Autodesk Fusion 360 part; units mm, degrees
(part 2 of 2)
sketch "Sketch4 (5)" plane through (0, 140, 0) normal (0, -1, 0) x (1, 0, 0) in component "Target holder left"
  line L0 (77, -34.8282) -> (74, -34.8282)
  line L1 (74, -34.8282) -> (74, -33.3282)
  line L2 (74, -33.3282) -> (77, -33.3282)
  line L3 (77, -33.3282) -> (77, -25.4282)
  line L4 (77, -25.4282) -> (62, -25.4282)
  line L5 (62, -25.4282) -> (62, -35.4282)
  line L6 (62, -35.4282) -> (77, -35.4282)
  line L7 (77, -35.4282) -> (77, -34.8282)
  line L8 (66.9731, -28.4282) -> (72.9731, -28.4282)
  line L9 (72.9731, -28.4282) -> (72.9731, -32.4282)
  line L10 (72.9731, -32.4282) -> (66.9731, -32.4282)
  line L11 (66.9731, -32.4282) -> (66.9731, -28.4282)
  line L12 (66.9731, -32.4282) -> (72.9731, -32.4282)
  line L13 (72.9731, -32.4282) -> (72.9731, -28.4282)
  line L14 (72.9731, -28.4282) -> (66.9731, -28.4282)
  line L15 (66.9731, -28.4282) -> (66.9731, -32.4282)
  constraint horizontal L12
  constraint vertical L13
  constraint horizontal L14
  constraint vertical L15
  constraint coincident L8.end L9.start
  constraint coincident L10.end L11.start
extrude "Extrude3''''''''" cut sketch "Sketch4 (5)" against normal blind 5 contours L8 L9 L10 L11 L12 L13 L14 L15 bodies 7 in component "Target holder left"
sketch "Sketch3 (8)" plane through (0, 140, 0) normal (0, -1, 0) x (1, 0, 0) in component "Target holder right"
  line L0 (243, -33.3282) -> (246, -33.3282)
  line L1 (246, -33.3282) -> (246, -34.8282)
  line L2 (246, -34.8282) -> (243, -34.8282)
  line L3 (243, -34.8282) -> (243, -35.4282)
  line L4 (243, -35.4282) -> (258, -35.4282)
  line L5 (258, -35.4282) -> (258, -25.4282)
  line L6 (258, -25.4282) -> (243, -25.4282)
  line L7 (243, -25.4282) -> (243, -33.3282)
  line L8 (246.9731, -28.4282) -> (252.9731, -28.4282)
  line L9 (252.9731, -28.4282) -> (252.9731, -32.4282)
  line L10 (252.9731, -32.4282) -> (246.9731, -32.4282)
  line L11 (246.9731, -32.4282) -> (246.9731, -28.4282)
  line L12 (246.9731, -28.4282) -> (252.9731, -28.4282)
  line L13 (252.9731, -28.4282) -> (252.9731, -32.4282)
  line L14 (252.9731, -32.4282) -> (246.9731, -32.4282)
  line L15 (246.9731, -32.4282) -> (246.9731, -28.4282)
  constraint horizontal L12
  constraint vertical L13
  constraint horizontal L14
  constraint vertical L15
  constraint coincident L9.end L10.start
  constraint coincident L8.start L11.end
extrude "Extrude3'''''''''" cut sketch "Sketch3 (8)" against normal blind 4 contours L8 L9 L10 L11 L12 L13 L14 L15 bodies 17 in component "Target holder right"
sketch "Sketch3 (9)" plane through (0, 0, -35.4282) normal (0, 0, -1) x (-1, 0, 0) in component "Target holder bottom"
  line L0 (-257.9731, 125.0758) -> (-61.9731, 125.0758)
  line L1 (-61.9731, 125.0758) -> (-61.9731, 140.0758)
  line L2 (-61.9731, 140.0758) -> (-257.9731, 140.0758)
  line L3 (-257.9731, 140.0758) -> (-257.9731, 125.0758)
  line L4 (-85.3026, 113.6358) -> (-67.6249, 131.3134)
  line L5 (-67.6249, 131.3134) -> (-77.5244, 141.2129)
  line L6 (-77.5244, 141.2129) -> (-95.2021, 123.5353)
  line L7 (-95.2021, 123.5353) -> (-85.3026, 113.6358)
  line L8 (-74.696, 138.3845) -> (-70.4534, 134.1419)
  line L9 (-70.4534, 134.1419) -> (-68.6856, 135.9096)
  line L10 (-68.6856, 135.9096) -> (-72.9282, 140.1523)
  line L11 (-72.9282, 140.1523) -> (-74.696, 138.3845)
  line L12 (-71.8676, 127.0708) -> (-81.06, 117.8784)
  line L13 (-81.06, 117.8784) -> (-79.2922, 116.1106)
  line L14 (-79.2922, 116.1106) -> (-70.0998, 125.303)
  line L15 (-70.0998, 125.303) -> (-71.8676, 127.0708)
  line L16 (-92.3737, 120.7068) -> (-88.131, 116.4642)
  line L17 (-88.131, 116.4642) -> (-89.8988, 114.6964)
  line L18 (-89.8988, 114.6964) -> (-94.1414, 118.9391)
  line L19 (-94.1414, 118.9391) -> (-92.3737, 120.7068)
  line L20 (-257.9731, 140.0758) -> (-257.9731, 125.0758)
  line L21 (-61.9731, 140.0758) -> (-257.9731, 140.0758)
  line L22 (-271.4131, 150.4053) -> (-253.7354, 132.7276)
  line L23 (-253.7354, 132.7276) -> (-243.8359, 142.6271)
  line L24 (-243.8359, 142.6271) -> (-261.5136, 160.3048)
  line L25 (-261.5136, 160.3048) -> (-271.4131, 150.4053)
  line L26 (-257.9731, 140.0758) -> (-257.9731, 136.9653)
  line L27 (-253.7354, 132.7276) -> (-257.9731, 136.9653)
  line L28 (-257.9731, 140.0758) -> (-246.3873, 140.0758)
  line L29 (-253.7354, 132.7276) -> (-246.3873, 140.0758)
  line L30 (-250.907, 135.5561) -> (-246.7408, 139.7222)
  line L31 (-246.7408, 139.7222) -> (-244.9731, 137.9545)
  line L32 (-244.9731, 137.9545) -> (-249.1392, 133.7883)
  line L33 (-249.1392, 133.7883) -> (-250.907, 135.5561)
  line L34 (-257.271, 136.2632) -> (-254.4425, 133.4348)
  line L35 (-254.4425, 133.4348) -> (-256.2103, 131.667)
  line L36 (-256.2103, 131.667) -> (-259.0387, 134.4954)
  line L37 (-259.0387, 134.4954) -> (-257.271, 136.2632)
  dimension "d197" = 2.5
  dimension "d198" = 2.5
  dimension "d199" = 2.5
  dimension "d200" = 4
  dimension "d201" = 4
  dimension "d202" = 6
  dimension "d203" = 6
  dimension "d204" = 4
  dimension "d205" = 4
  dimension "d221" = 2.5
  dimension "d222" = 4
  dimension "d223" = 0.5
  dimension "d238" = 2.5
  dimension "d239" = 1
  dimension "d240" = 4
  constraint perpendicular L8 L9
  constraint parallel L8 L10
  constraint parallel L9 L11
  constraint coincident L5 L8.end
  constraint coincident L5 L8.start
  constraint perpendicular L12 L13
  constraint parallel L12 L14
  constraint parallel L13 L15
  constraint coincident L4 L12.end
  constraint perpendicular L5 L12
  constraint perpendicular L16 L17
  constraint parallel L16 L18
  constraint parallel L17 L19
  constraint coincident L7 L16.end
  constraint perpendicular L14 L16
  constraint coincident L21 L28.end
  constraint coincident L23 L28.end
  constraint coincident L2.end L3.start
  constraint coincident L22 L26.end
  constraint coincident L20 L26.end
  constraint coincident L22.end L23.start
  constraint perpendicular L30 L31
  constraint parallel L30 L32
  constraint parallel L31 L33
  constraint coincident L23 L30.end
  constraint parallel L23 L30
  constraint perpendicular L34 L35
  constraint parallel L34 L36
  constraint parallel L35 L37
  constraint coincident L22 L34.end
  constraint parallel L22 L34
  measures "d197" distance of L8.end L9.end
  measures "d198" distance of L12.start L14.end
  measures "d199" distance of L16.end L17.end
  measures "d200" distance of L6.end L16.start
  measures "d201" distance of L4.start L16.end
  measures "d202" distance of L4.start L12.end
  measures "d203" distance of L4.end L12.start
  measures "d204" distance of L4.end L8.end
  measures "d205" distance of L5.end L8.start
  measures "d221" distance of L30.start L32.end
  measures "d222" distance of L22.end L30.start
  measures "d223" distance of L28.end L30.end
  measures "d238" distance of L34.end L35.end
  measures "d239" distance of L22.end L34.end
  measures "d240" distance of L34.start L34.end
extrude "Extrude8" add sketch "Sketch3 (9)" along normal blind 12 contours L0 L4 L12 L14 L15 | L0 L4 L12 L13 L14 | L7 L16 L17 L18 L19 | L2 L10 L11 L21 | L2 L5 L8 L9 L10 L11 L21 bodies 16 makes body 18 at (90.9595, 119.2926, -43.4282) in component "Target holder bottom"
extrude "Extrude10" add sketch "Sketch3 (9)" along normal blind 12 contours L3 L20 L22 L27 L34 L35 L36 L37 | L23 L29 L30 L31 L32 L33 bodies 16 in component "Target holder bottom"
extrude "Extrude11" add sketch "Sketch3 (9)" against normal blind 2 contours L0 L4 L6 L7 L12 L16 | L0 L4 L12 L13 L14 | L7 L16 L17 L18 L19 bodies 16 18 in component "Target holder bottom"
sketch "Sketch4 (6)" plane through (0, 0, -35.4282) normal (0, 0, -1) x (-1, 0, 0) in component "Target holder right"
  line L0 (-243, 310) -> (-258, 310)
  line L1 (-258, 310) -> (-258, 140)
  line L2 (-258, 140) -> (-243, 140)
  line L3 (-243, 140) -> (-243, 310)
  line L4 (-271.4131, 150.4053) -> (-253.7354, 132.7276)
  line L5 (-253.7354, 132.7276) -> (-243.8359, 142.6271)
  line L6 (-243.8359, 142.6271) -> (-261.5136, 160.3048)
  line L7 (-261.5136, 160.3048) -> (-271.4131, 150.4053)
  line L8 (-258, 156.7912) -> (-261.5136, 160.3048)
  line L9 (-261.5136, 160.3048) -> (-271.4131, 150.4053)
  line L10 (-258, 140) -> (-261.0078, 140)
  line L11 (-261.0078, 140) -> (-271.4131, 150.4053)
  line L12 (-258, 140) -> (-258, 156.7912)
  line L13 (-264.342, 157.4764) -> (-268.5847, 153.2337)
  line L14 (-268.5847, 153.2337) -> (-270.3524, 155.0015)
  line L15 (-270.3524, 155.0015) -> (-266.1098, 159.2442)
  line L16 (-266.1098, 159.2442) -> (-264.342, 157.4764)
  line L17 (-267.1705, 146.1627) -> (-261.3613, 140.3536)
  line L18 (-261.3613, 140.3536) -> (-263.1291, 138.5858)
  line L19 (-263.1291, 138.5858) -> (-268.9382, 144.3949)
  line L20 (-268.9382, 144.3949) -> (-267.1705, 146.1627)
  line L21 (-234.6436, 336.5158) -> (-252.3212, 318.8382)
  line L22 (-252.3212, 318.8382) -> (-242.4217, 308.9387)
  line L23 (-242.4217, 308.9387) -> (-224.7441, 326.6163)
  line L24 (-224.7441, 326.6163) -> (-234.6436, 336.5158)
  line L25 (-258, 310) -> (-252.3212, 318.8382)
  line L26 (-252.3212, 318.8382) -> (-234.6436, 336.5158)
  line L27 (-234.6436, 336.5158) -> (-224.7441, 326.6163)
  line L28 (-243, 310) -> (-241.3604, 310)
  line L29 (-241.3604, 310) -> (-224.7441, 326.6163)
  line L30 (-248.0786, 323.0808) -> (-238.8862, 332.2732)
  line L31 (-238.8862, 332.2732) -> (-240.654, 334.0409)
  line L32 (-240.654, 334.0409) -> (-249.8464, 324.8486)
  line L33 (-249.8464, 324.8486) -> (-248.0786, 323.0808)
  line L34 (-249.4928, 316.0097) -> (-245.2502, 311.7671)
  line L35 (-245.2502, 311.7671) -> (-247.0179, 309.9993)
  line L36 (-247.0179, 309.9993) -> (-251.2606, 314.242)
  line L37 (-251.2606, 314.242) -> (-249.4928, 316.0097)
  line L38 (-231.8151, 333.6874) -> (-227.5725, 329.4448)
  line L39 (-227.5725, 329.4448) -> (-225.8047, 331.2125)
  line L40 (-225.8047, 331.2125) -> (-230.0474, 335.4552)
  line L41 (-230.0474, 335.4552) -> (-231.8151, 333.6874)
  dimension "d228" = 2.5
  dimension "d229" = 2.5
  dimension "d230" = 4
  dimension "d231" = 4
  dimension "d232" = 6
  dimension "d233" = 0.5
  dimension "d254" = 2.5
  dimension "d255" = 6
  dimension "d256" = 6
  dimension "d257" = 2.5
  dimension "d258" = 4
  dimension "d259" = 4
  dimension "d261" = 2.5
  dimension "d262" = 4
  dimension "d263" = 4
  constraint coincident L1 L8.start
  constraint coincident L6 L8.start
  constraint coincident L6.end L7.start
  constraint coincident L4.start L7.end
  constraint coincident L1.end L2.start
  constraint coincident L4 L10.end
  constraint perpendicular L1 L10
  constraint perpendicular L13 L14
  constraint parallel L13 L15
  constraint parallel L14 L16
  constraint coincident L7 L13.end
  constraint parallel L7 L13
  constraint perpendicular L17 L18
  constraint parallel L17 L19
  constraint parallel L18 L20
  constraint coincident L11 L17.end
  constraint perpendicular L9 L17
  constraint coincident L0.end L1.start
  constraint coincident L21.end L22.start
  constraint coincident L21.start L24.end
  constraint coincident L23.end L24.start
  constraint coincident L0.start L3.end
  constraint coincident L23 L28.end
  constraint perpendicular L3 L28
  constraint perpendicular L30 L31
  constraint parallel L30 L32
  constraint parallel L31 L33
  constraint coincident L21 L30.end
  constraint parallel L21 L30
  constraint perpendicular L34 L35
  constraint parallel L34 L36
  constraint parallel L35 L37
  constraint coincident L22 L34.end
  constraint perpendicular L26 L34
  constraint perpendicular L38 L39
  constraint parallel L38 L40
  constraint parallel L39 L41
  constraint coincident L27 L38.end
  constraint perpendicular L35 L38
  measures "d228" distance of L13.end L14.end
  measures "d229" distance of L17.start L19.end
  measures "d230" distance of L4.start L13.end
  measures "d231" distance of L6.end L13.start
  measures "d232" distance of L4.start L17.start
  measures "d233" distance of L10.end L17.end
  measures "d254" distance of L30.start L32.end
  measures "d255" distance of L21.end L30.start
  measures "d256" distance of L21.start L30.end
  measures "d257" distance of L38.start L40.end
  measures "d258" distance of L21.start L38.start
  measures "d259" distance of L23.end L38.end
  measures "d261" distance of L34.start L36.end
  measures "d262" distance of L21.end L34.start
  measures "d263" distance of L22.end L34.end
extrude "Extrude4''''''''" add sketch "Sketch4 (6)" along normal blind 12 separate body contours L7 L9 L13 L14 L15 L16 | L4 L11 L17 L18 L19 L20 makes body 19 at (268.9382, 156.4157, -39.4282) makes body 20 at (265.2341, 144.2263, -39.4282) in component "Target holder right"
extrude "Extrude5'" add sketch "Sketch4 (6)" against normal blind 2 contours L1 L4 L6 L7 L8 L9 L10 L11 L12 L13 L17 | L7 L9 L13 L14 L15 L16 | L4 L11 L17 L18 L19 L20 bodies 17 19 20 in component "Target holder right"
sketch "Sketch5" plane through (0, 0, -35.4282) normal (0, 0, -1) x (-1, 0, 0) in component "Target holder left"
  line L0 (-62, 310) -> (-77, 310)
  line L1 (-77, 310) -> (-77, 140)
  line L2 (-77, 140) -> (-62, 140)
  line L3 (-62, 140) -> (-62, 310)
  line L4 (-48.533, 299.7463) -> (-66.2107, 317.4239)
  line L5 (-66.2107, 317.4239) -> (-76.1102, 307.5244)
  line L6 (-76.1102, 307.5244) -> (-58.4325, 289.8468)
  line L7 (-58.4325, 289.8468) -> (-48.533, 299.7463)
  line L8 (-73.2818, 310.3529) -> (-69.0391, 314.5955)
  line L9 (-69.0391, 314.5955) -> (-70.8069, 316.3633)
  line L10 (-70.8069, 316.3633) -> (-75.0496, 312.1206)
  line L11 (-75.0496, 312.1206) -> (-73.2818, 310.3529)
  line L12 (-61.9681, 313.1813) -> (-52.7757, 303.9889)
  line L13 (-52.7757, 303.9889) -> (-51.0079, 305.7567)
  line L14 (-51.0079, 305.7567) -> (-60.2003, 314.9491)
  line L15 (-60.2003, 314.9491) -> (-61.9681, 313.1813)
  line L16 (-51.3615, 296.9178) -> (-55.6041, 292.6752)
  line L17 (-55.6041, 292.6752) -> (-53.8364, 290.9074)
  line L18 (-53.8364, 290.9074) -> (-49.5937, 295.1501)
  line L19 (-49.5937, 295.1501) -> (-51.3615, 296.9178)
  line L20 (-66.2107, 317.4239) -> (-48.533, 299.7463)
  line L21 (-48.533, 299.7463) -> (-58.4325, 289.8468)
  line L22 (-58.4325, 289.8468) -> (-62, 293.4142)
  line L23 (-62, 293.4142) -> (-62, 310)
  line L24 (-73.6347, 310) -> (-73.2818, 310.3529)
  line L25 (-73.6347, 310) -> (-62, 310)
  dimension "d241" = 2.5
  dimension "d242" = 4
  dimension "d243" = 4
  dimension "d244" = 2.5
  dimension "d245" = 6
  dimension "d246" = 6
  dimension "d247" = 2.5
  dimension "d248" = 4
  dimension "d249" = 4
  constraint perpendicular L8 L9
  constraint parallel L8 L10
  constraint parallel L9 L11
  constraint coincident L5 L8.end
  constraint coincident L5 L8.start
  constraint perpendicular L12 L13
  constraint parallel L12 L14
  constraint parallel L13 L15
  constraint coincident L4 L12.end
  constraint perpendicular L5 L12
  constraint perpendicular L16 L17
  constraint parallel L16 L18
  constraint parallel L17 L19
  constraint coincident L7 L16.end
  constraint perpendicular L4 L16
  constraint coincident L4.end L5.start
  constraint coincident L4.start L7.end
  constraint coincident L6.end L7.start
  constraint coincident L3 L22.end
  constraint coincident L6 L22.end
  constraint coincident L0.start L3.end
  constraint coincident L0 L24.start
  constraint coincident L5 L24.start
  measures "d241" distance of L8.start L10.end
  measures "d242" distance of L5.end L8.start
  measures "d243" distance of L4.end L8.end
  measures "d244" distance of L12.start L14.end
  measures "d245" distance of L4.end L12.start
  measures "d246" distance of L4.start L12.end
  measures "d247" distance of L16.start L18.end
  measures "d248" distance of L4.start L16.start
  measures "d249" distance of L6.end L16.end
extrude "Extrude4'''''''''" add sketch "Sketch5" along normal blind 12 separate body contours L5 L8 L9 L10 L11 | L7 L16 L17 L18 L19 L21 | L4 L12 L13 L14 L15 L20 makes body 21 at (70.4534, 313.1813, -39.4282) makes body 22 at (54.0721, 308.8208, -39.4282) makes body 23 at (54.1899, 294.0894, -39.4282) in component "Target holder left"
extrude "Extrude5''" add sketch "Sketch5" against normal blind 2 contours L0 L3 L4 L5 L6 L7 L8 L12 L16 L20 L21 L22 L23 L24 L25 | L5 L8 L9 L10 L11 | L7 L16 L17 L18 L19 L21 | L4 L12 L13 L14 L15 L20 bodies 7 21 22 23 in component "Target holder left"
extrude "Extrude6'" add sketch "Sketch4 (6)" along normal blind 12 separate body contours L22 L34 L35 L36 L37 | L21 L26 L30 L31 L32 L33 | L24 L27 L38 L39 L40 L41 makes body 24 at (227.2189, 332.6267, -39.4282) makes body 25 at (241.9503, 329.2091, -39.4282) makes body 26 at (248.4321, 311.4135, -39.4282) in component "Target holder right"
extrude "Extrude7'" add sketch "Sketch4 (6)" against normal blind 2 contours L0 L22 L35 | L22 L34 L35 L36 L37 | L0 L22 L25 L36 L37 | L0 L21 L22 L23 L24 L26 L27 L28 L29 L30 L34 L38 | L21 L26 L30 L31 L32 L33 | L24 L27 L38 L39 L40 L41 bodies 17 24 25 26 in component "Target holder right"
sketch "Sketch5 (2)" plane through (243, 0, 0) normal (-1, 0, 0) x (0, 0, 1) in component "Target holder right"
  line L0 (-33.3282, 310) -> (-33.3282, 140)
  line L1 (-33.3282, 140) -> (-25.4282, 140)
  line L2 (-25.4282, 140) -> (-25.4282, 310)
  line L3 (-25.4282, 310) -> (-33.3282, 310)
  line L4 (-33.3282, 310) -> (-33.3282, 302)
  line L5 (-33.3282, 302) -> (-29.3282, 310)
  line L6 (-29.3282, 310) -> (-33.3282, 310)
  dimension "d268" = 8
  dimension "d269" = 4
  constraint coincident L0.start L3.end
  constraint coincident L0 L4.end
  constraint parallel L0 L4
  constraint coincident L3 L5.end
  measures "d268" distance of L4.end L0.start
  measures "d269" distance of L5.end L0.start
extrude "Extrude8'" cut sketch "Sketch5 (2)" against normal up to surface (3 mm away) contours L0 L3 L4 L5 L6 bodies 17 in component "Target holder right"
sketch "Sketch6" plane through (77, 0, 0) normal (1, 0, 0) x (0, 0, -1) in component "Target holder left"
  line L0 (33.3282, 140) -> (33.3282, 310)
  line L1 (33.3282, 310) -> (25.4282, 310)
  line L2 (25.4282, 310) -> (25.4282, 140)
  line L3 (25.4282, 140) -> (33.3282, 140)
  line L4 (33.3282, 310) -> (33.3282, 302)
  line L5 (33.3282, 302) -> (29.3782, 310)
  line L6 (29.3782, 310) -> (33.3282, 310)
  dimension "d272" = 8
  constraint coincident L0.end L1.start
  constraint coincident L0 L4.end
  constraint perpendicular L1 L4
  constraint midpoint L1 L5.end
  measures "d272" distance of L0.end L4.end
extrude "Extrude6''" cut sketch "Sketch6" against normal up to surface (3 mm away) contours L0 L1 L4 L5 L6 bodies 7 in component "Target holder left"
component "Bottom holder OLD" placed x (1, 0, 0) y (0, 1, 0) z (0, 0, 1) at (0, 0, 0)
component "Left holder OLD" placed x (1, 0, 0) y (0, 1, 0) z (0, 0, 1) at (0, 0, 0)
component "Right holder OLD" placed x (1, 0, 0) y (0, 1, 0) z (0, 0, 1) at (0, 0, 0)
component "Faceplate" placed x (1, 0, 0) y (0, 1, 0) z (0, 0, 1) at (0, 0, 0)
component "Backplate" placed x (1, 0, 0) y (0, 1, 0) z (0, 0, 1) at (-0.0957, 0.2508, -0.8034)
component "Sensor-Holder West" placed x (1, 0, 0) y (0, 1, 0) z (0, 0, 1) at (-2.7704, -3.6866, 0.0718)
component "Help lines" placed x (1, 0, 0) y (0, 1, 0) z (0, 0, 1) at (-0.0269, 0.0758, 0.0718)
component "Sensor-Holder South" placed x (0, 1, 0) y (-1, 0, 0) z (0, 0, 1) at (388.7354, 62.3323, 0.0718)
component "Sensor-Holder North" placed x (0, -1, 0) y (1, 0, 0) z (0, 0, 1) at (-68.7893, 387.8193, 0.0718)
component "Sensor-Holder East" placed x (-1, 0, 0) y (0, -1, 0) z (0, 0, 1) at (322.7166, 453.8382, 0.0718)
component "Target holder bottom" placed x (1, 0, 0) y (0, 1, 0) z (0, 0, 1) at (0, 0, 0)
component "Target holder right" placed x (1, 0, 0) y (0, 1, 0) z (0, 0, 1) at (0, 0, 0)
component "Target holder left" placed x (1, 0, 0) y (0, 1, 0) z (0, 0, 1) at (0, 0, 0)
component "Sensor West" placed x (1, 0, 0) y (0, 1, 0) z (0, 0, 1) at (0, 0, 0) in component "Sensor-Holder West"
component "Sensor South" placed x (1, 0, 0) y (0, 1, 0) z (0, 0, 1) at (0, 0, 0) in component "Sensor-Holder South"
component "Sensor North" placed x (1, 0, 0) y (0, 1, 0) z (0, 0, 1) at (0, 0, 0) in component "Sensor-Holder North"
component "Sensor West (1)" placed x (1, 0, 0) y (0, 1, 0) z (0, 0, 1) at (0, 0, 0) in component "Sensor-Holder East"
